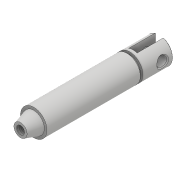
# Autodesk Inventor part: kern
Saved by Autodesk Inventor 2018.1 (Build 221171000, 171)
## iProperties
Created: 2019-06-27
Part Number: kern
Material: Типовые
Document SubType Name: Modeling
Designer: Boss
Mass: 1.7372 g
Surface Area: 13.1028 cm^2
Volume: 1.7372 cm^3
Density: 1 g/cm^3
Appearance: По умолчанию
Author: Boss
Autodesk Inventor part; units mm, degrees
ref_plane "YZ Plane" through (0, 0, 0) normal (1, 0, 0) x (0, 1, 0)
ref_plane "XZ Plane" through (0, 0, 0) normal (0, 1, 0) x (-1, 0, 0)
ref_plane "XY Plane" through (0, 0, 0) normal (0, 0, 1) x (1, 0, 0)
sketch "Эскиз1" plane through (0, 0, 0) normal (0, 0, 1) x (1, 0, 0)
  line L0 (0, 0) -> (0, 50)
  line L1 (0, 42) -> (4, 42)
  line L2 (4, 42) -> (4, 33)
  line L3 (4, 33) -> (3.2, 33)
  line L4 (3.2, 33) -> (3.2, 32.2)
  line L5 (3.2, 32.2) -> (4, 32.2)
  line L6 (4, 32.2) -> (4, 4)
  line L7 (4, 4) -> (3.2, 4)
  line L8 (2, 0) -> (0, 0)
  line L9 (3.2, 4) -> (2, 0)
  dimension "d0" = 50
  dimension "d1" = 42
  dimension "d2" = 8
  dimension "d3" = 0.8
  dimension "d4" = 2
  dimension "d5" = 4
  dimension "d6" = 0.8
  dimension "d7" = 9
  constraints: 20 end point, 4 point on line, 2 equal length, 1 collinear, 1 perpendicular, 1 vertical
  measures "d0" distance of L0.start L0.end
  measures "d1" distance between parallel lines of L8 L1
  measures "d2" diameter of L6 L0
  measures "d3" distance between parallel lines of L2 L4
  measures "d4" distance of L8.start L8.end
  measures "d5" distance between parallel lines of L8 L7
  measures "d6" distance of L6.end L7.end
  measures "d7" distance of L1.end L2.end
revolve "Вращение1" add sketch "Эскиз1" angle 360 about axis through (0, 0, 0) along (0, 1, 0)
hole "Отверстие1" at (0, 0, 0) direction (0, 1, 0) diameter 2.459 depth 10 tip angle 118 thread size "M3x0.5" class "6H" standard "ANSI Metric M Profile"
chamfer "Фаска1" distance 0.1 angle 45 1 edges at (-4, 42, 0)
sketch "Эскиз2" plane through (0, 42, 0) normal (0, 1, 0) x (1, 0, 0)
  circle A0 centre (0, 0) radius 3.9 projected
  line L0 (1.25, 4.0963) -> (-1.25, 4.0963)
  line L1 (-1.25, 4.0963) -> (-1.25, -4.0963)
  line L2 (-1.25, -4.0963) -> (1.25, -4.0963)
  line L3 (1.25, -4.0963) -> (1.25, 4.0963)
  line L4 (1.25, 4.0963) -> (-1.25, -4.0963) construction
  line L5 (-1.25, 4.0963) -> (1.25, -4.0963) construction
  dimension "d23" = 2.5
  constraints: 12 end point, 2 midpoint
  measures "d23" distance of L2.end L1.end
extrude "Выдавливание1" cut sketch "Эскиз2" against normal blind 8 contours L3 A0 L1 | A0 L1 L0 L3 | L3 L2 L1 A0
hole "Отверстие2" at (-1.25, 39, 0.2003) direction (-1, 0, 0) diameter 3 end through all both
chamfer "Фаска2" distance 0.3 angle 45 4 edges at (-3.6206, 39.0021, 1.7003) (3.8791, 39.9309, -0.9759) (3.8791, 38.0692, -0.9759) (3.6206, 38.9989, 1.7003)
